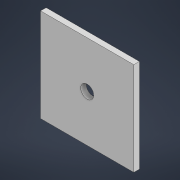
# Autodesk Inventor part: arm2
Saved by Autodesk Inventor 2021 (Build 250183000, 183)
## iProperties
Created: 2022-05-25
Part Number: arm2
Material: Generic
Document SubType Name: Modeling
Designer: techv
Density: 1 g/cm^3
Appearance: Default
Author: techv
Autodesk Inventor part; units mm, degrees
ref_plane "YZ Plane" through (0, 0, 0) normal (1, 0, 0) x (0, 1, 0)
ref_plane "XZ Plane" through (0, 0, 0) normal (0, 1, 0) x (-1, 0, 0)
ref_plane "XY Plane" through (0, 0, 0) normal (0, 0, 1) x (1, 0, 0)
sketch "Sketch1" plane through (0, 0, 0) normal (0, 0, 1) x (1, 0, 0)
  ellipse E0 centre (0, 0) end of major axis (0, 3.5) minor radius 3.5 projected
  arc A0 (-2.0076, 1.85) -> (-2.0076, -1.85) centre (0, 0) ccw projected
  line L0 (-2.0076, 1.85) -> (2.0076, 1.85) projected
  arc A1 (2.0076, -1.85) -> (2.0076, 1.85) centre (0, 0) ccw projected
  line L1 (2.0076, -1.85) -> (-2.0076, -1.85) projected
  line L2 (-50, -25) -> (50, -25)
  line L3 (50, -25) -> (50, 25)
  line L4 (50, 25) -> (-50, 25)
  line L5 (-50, 25) -> (-50, -25)
  line L6 (-50, -25) -> (50, 25) construction
  line L7 (50, -25) -> (-50, 25) construction
  line L8 (-25, -25) -> (-25, 25)
  line L9 (25, -25) -> (25, 25)
  point P0 (0, 0)
  dimension "d0" = 100
  dimension "d1" = 50
  dimension "d4" = 25
  dimension "d5" = 50
  constraints: 16 end point, 4 point on line, 3 perpendicular, 2 midpoint, 2 parallel, 1 horizontal, 1 other
  measures "d0" distance of L4.end L3.end
  measures "d1" distance of L3.end L2.end
  measures "d4" distance between parallel lines of L3 L9
  measures "d5" distance between parallel lines of L8 L9
extrude "Extrusion1" add sketch "Sketch1" against normal blind 3 contours L8 L4 L9 L2
body "Solid1"
